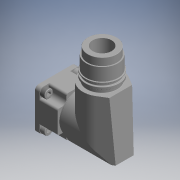
# Autodesk Inventor part: SCHUNK-Stecker ERD
Saved by Autodesk Inventor 2017.3 (Build 213256000, 256)
## iProperties
Part Number: SCHUNK-Stecker ERD
Material: Generic
Catalog Web Link: www.cadenas.de
Description: Connector-Miniature rotary unit
Vendor: SCHUNK
Document SubType Name: Modeling
Designer: partserver
Manufacturer: SCHUNK
Mass: 19.4018 g
Surface Area: 56.9329 cm^2
Volume: 19.4018 cm^3
Density: 1 g/cm^3
Appearance: PSOLRGB-192-192-192
Category: PARTsolutions
Company: SCHUNK
Title: SCHUNK-Stecker ERD
Author: Cadenas PARTsolutions
Comments: Miniature rotary unit
PSOL_IDENT_0: {$CADENAS_DATA\23d-libs\schunk\greifsysteme\drehmodule\drehmodule_elektrisch\schwenkeinheiten\miniat
PSOL_IDENT_1: ur_schwenkeinheiten\erd_stk.prj},179 {VTYP=3D},{NB=SCHUNK-Stecker ERD},{LINA=SCHUNK-Stecker ERD},{NN=
PSOL_IDENT_2: Connector},{DATE=23.04.2020 15:23:31},{GEOMDATE=04.12.2019 08:06:04},{VERSION=},{LINEID=10},{WBVAR=}
PSOL_IDENT_3: ,{WBNUMERIC=}  {NB=SCHUNK-Stecker ERD},{LINA=SCHUNK-Stecker ERD},{KT=DUMMY},{TYP=ERD}
NB: SCHUNK-Stecker ERD
NN: Connector
NT: Miniature rotary unit
NBSYN: SCHUNK-Stecker $TYP.
LINA: SCHUNK-Stecker ERD
CATALOG: SCHUNK
TYP: ERD
SUPPLIER: SCHUNK
ARTICLENO: SCHUNK-Stecker ERD
BOMINFO: SCHUNK-Stecker ERD
CREATOR: CADENAS GmbH
Autodesk Inventor part; units mm, degrees
sketch "Sketch_7" plane through (0, 0, 0) normal (1, 0, 0) x (0, 1, 0)
  line L0 (21.3, -2.9) -> (3.7, -2.9)
  arc A0 (3.7, -2.9) -> (1.7, -4.9) centre (3.7, -4.9) ccw
  line L1 (1.7, -4.9) -> (1.7, -22.5)
  arc A1 (1.7, -22.5) -> (3.7, -24.5) centre (3.7, -22.5) ccw
  line L2 (3.7, -24.5) -> (21.3, -24.5)
  arc A2 (21.3, -24.5) -> (23.3, -22.5) centre (21.3, -22.5) ccw
  line L3 (23.3, -22.5) -> (23.3, -4.9)
  arc A3 (23.3, -4.9) -> (21.3, -2.9) centre (21.3, -4.9) ccw
  constraints: 8 end point, 8 point on circle, 4 centre point
extrude "Extrusion1" add sketch "Sketch_7" against normal blind 12
sketch "Sketch_8" plane through (-12, 0, 0) normal (1, 0, 0) x (0, 0, -1)
  line L0 (0.9, -0.3) -> (26.5, -0.3)
  line L1 (26.5, -0.3) -> (26.5, 25.3)
  line L2 (26.5, 25.3) -> (0.9, 25.3)
  line L3 (0.9, 25.3) -> (0.9, -0.3)
  arc A0 (2.9, 7.4) -> (3.9, 6.4) centre (3.9, 7.4) ccw
  line L4 (3.9, 6.4) -> (5.3, 6.4)
  arc A1 (7.6, 4.1) -> (5.3, 6.4) centre (5.3, 4.1) ccw
  line L5 (7.6, 4.1) -> (7.6, 2.7)
  arc A2 (7.6, 2.7) -> (8.6, 1.7) centre (8.6, 2.7) ccw
  line L6 (8.6, 1.7) -> (18.8, 1.7)
  arc A3 (18.8, 1.7) -> (19.8, 2.7) centre (18.8, 2.7) ccw
  line L7 (19.8, 2.7) -> (19.8, 4.1)
  arc A4 (22.1, 6.4) -> (19.8, 4.1) centre (22.1, 4.1) ccw
  line L8 (22.1, 6.4) -> (23.5, 6.4)
  arc A5 (23.5, 6.4) -> (24.5, 7.4) centre (23.5, 7.4) ccw
  line L9 (24.5, 7.4) -> (24.5, 17.6)
  arc A6 (24.5, 17.6) -> (23.5, 18.6) centre (23.5, 17.6) ccw
  line L10 (23.5, 18.6) -> (22.1, 18.6)
  arc A7 (19.8, 20.9) -> (22.1, 18.6) centre (22.1, 20.9) ccw
  line L11 (19.8, 20.9) -> (19.8, 22.3)
  arc A8 (19.8, 22.3) -> (18.8, 23.3) centre (18.8, 22.3) ccw
  line L12 (18.8, 23.3) -> (8.6, 23.3)
  arc A9 (8.6, 23.3) -> (7.6, 22.3) centre (8.6, 22.3) ccw
  line L13 (7.6, 22.3) -> (7.6, 20.9)
  arc A10 (5.3, 18.6) -> (7.6, 20.9) centre (5.3, 20.9) ccw
  line L14 (5.3, 18.6) -> (3.9, 18.6)
  arc A11 (3.9, 18.6) -> (2.9, 17.6) centre (3.9, 17.6) ccw
  line L15 (2.9, 17.6) -> (2.9, 7.4)
  constraints: 32 end point, 24 point on circle, 12 centre point
extrude "Extrusion2" cut sketch "Sketch_8" along normal blind 9.5
sketch "Sketch_9" plane through (0, 0, -13.7) normal (0, 0, 1) x (1, 0, 0)
  line L0 (50, 12.5) -> (-50, 12.5)
  line L1 (-36.93, 12.5) -> (-36.93, 22.75)
  line L2 (-36.93, 22.75) -> (-12.75, 22.75)
  arc A0 (-12.75, 22.75) -> (-12.35, 22.35) centre (-12.35, 22.75) ccw
  line L3 (-12.35, 22.35) -> (-12, 22.35)
  line L4 (-12, 22.35) -> (-12, 12.5)
  line L5 (-12, 12.5) -> (-36.93, 12.5)
  constraints: 12 end point, 2 point on circle, 1 centre point
revolve "Revolution1" add sketch "Sketch_9" angle 360 about axis through (50, 12.5, -13.7) along (1, 0, 0)
sketch "Sketch_10" plane through (-36.93, 0, 0) normal (1, 0, 0) x (0, 0, -1)
  line L0 (3.3, 18.15) -> (3.3, 6.85)
  line L1 (3.3, 6.85) -> (8.5222, 3.7133)
  line L2 (8.5222, 3.7133) -> (8.5222, 21.2867)
  line L3 (8.5222, 21.2867) -> (3.3, 18.15)
  constraints: 8 end point
extrude "Extrusion3" add sketch "Sketch_10" along normal blind 24.18
sketch "Sketch_11" plane through (-24.8327, 0, 0) normal (1, 0, 0) x (0, 0, -1)
  line L0 (50.05, 12.5) -> (13.7, 12.5)
  line L1 (13.7, 12.5) -> (13.7, 22.75)
  line L2 (13.7, 22.75) -> (33.95, 22.75)
  line L3 (33.95, 22.75) -> (33.95, 20.65)
  arc A0 (33.95, 20.65) -> (34.1, 20.5) centre (34.1, 20.65) ccw
  line L4 (34.1, 20.5) -> (36.05, 20.5)
  line L5 (36.05, 20.5) -> (36.05, 21.35)
  arc A1 (36.2, 21.5) -> (36.05, 21.35) centre (36.2, 21.35) ccw
  line L6 (36.2, 21.5) -> (37.2, 21.5)
  arc A2 (37.35, 21.35) -> (37.2, 21.5) centre (37.2, 21.35) ccw
  line L7 (37.35, 21.35) -> (37.35, 20.75)
  arc A3 (37.35, 20.75) -> (37.5, 20.6) centre (37.5, 20.75) ccw
  line L8 (37.5, 20.6) -> (38.7, 20.6)
  arc A4 (38.7, 20.6) -> (38.85, 20.75) centre (38.7, 20.75) ccw
  line L9 (38.85, 20.75) -> (38.85, 21.35)
  arc A5 (39, 21.5) -> (38.85, 21.35) centre (39, 21.35) ccw
  line L10 (39, 21.5) -> (39.3, 21.5)
  arc A6 (39.45, 21.35) -> (39.3, 21.5) centre (39.3, 21.35) ccw
  line L11 (39.45, 21.35) -> (39.45, 20.9)
  line L12 (39.45, 20.9) -> (46.15, 20.9)
  line L13 (46.15, 20.9) -> (46.15, 20.25)
  line L14 (46.15, 20.25) -> (49.9, 20.25)
  arc A7 (50.05, 20.1) -> (49.9, 20.25) centre (49.9, 20.1) ccw
  line L15 (50.05, 20.1) -> (50.05, 17.5)
  line L16 (50.05, 17.5) -> (42.05, 17.5)
  line L17 (42.05, 17.5) -> (42.05, 12.5)
  line L18 (42.05, 12.5) -> (13.7, 12.5)
  constraints: 38 end point, 16 point on circle, 8 centre point
revolve "Revolution2" add sketch "Sketch_11" angle 360 about axis through (-24.8327, 12.5, -50.05) along (0, 0, -1)
sketch "Sketch_13" plane through (0, 0, -13.7) normal (0, 0, 1) x (1, 0, 0)
  line L0 (-36.8327, 17.249) -> (-36.8327, 7.751)
  line L1 (-36.8327, 7.751) -> (-30.1105, 3.7133)
  line L2 (-30.1105, 3.7133) -> (-30.1105, 21.2867)
  line L3 (-30.1105, 21.2867) -> (-36.8327, 17.249)
  constraints: 8 end point
extrude "Extrusion4" add sketch "Sketch_13" against normal blind 20.25
sketch "Sketch_12" plane through (0, 0, -3.2) normal (0, 0, 1) x (1, 0, 0)
  line L0 (-39.8327, -0.15) -> (-24.8327, -0.15)
  line L1 (-24.8327, -0.15) -> (-24.8327, 2.25)
  arc A0 (-30.1105, 3.7133) -> (-24.8327, 2.25) centre (-24.8327, 12.5) ccw
  line L2 (-30.1105, 3.7133) -> (-36.8327, 7.751)
  line L3 (-36.8327, 7.751) -> (-36.8327, 17.249)
  line L4 (-36.8327, 17.249) -> (-30.1105, 21.2867)
  arc A1 (-24.8327, 22.75) -> (-30.1105, 21.2867) centre (-24.8327, 12.5) ccw
  line L5 (-24.8327, 22.75) -> (-24.8327, 25.15)
  line L6 (-24.8327, 25.15) -> (-39.8327, 25.15)
  line L7 (-39.8327, 25.15) -> (-39.8327, -0.15)
  constraints: 16 end point, 4 point on circle, 2 centre point
extrude "Extrusion5" cut sketch "Sketch_12" against normal blind 30.6878
sketch "Sketch_14" plane through (0, 0, 0) normal (0, 1, 0) x (-1, 0, 0)
  line L0 (36.833, -43.1878) -> (36.833, -2.25)
  line L1 (36.833, -2.25) -> (34.0601, -43.1878)
  line L2 (34.0601, -43.1878) -> (36.833, -43.1878)
  constraints: 6 end point
extrude "Extrusion6" cut sketch "Sketch_14" along normal blind 30.25
sketch "Sketch_31" plane through (0, 0, -5.3) normal (0, 0, 1) x (1, 0, 0)
  line L0 (50, 20.9) -> (-50, 20.9)
  line L1 (-5, 20.9) -> (-5, 22.85)
  arc A0 (-4.7, 23.15) -> (-5, 22.85) centre (-4.7, 22.85) ccw
  line L2 (-4.7, 23.15) -> (-2.5, 23.15)
  line L3 (-2.5, 23.15) -> (-2.5, 20.9)
  line L4 (-2.5, 20.9) -> (-5, 20.9)
  constraints: 10 end point, 2 point on circle, 1 centre point
revolve "Revolution3" add sketch "Sketch_31" angle 360 about axis through (50, 20.9, -5.3) along (1, 0, 0)
sketch "Sketch_32" plane through (0, 0, -5.3) normal (0, 0, 1) x (1, 0, 0)
  line L0 (50, 4.1) -> (-50, 4.1)
  line L1 (-5, 4.1) -> (-5, 6.05)
  arc A0 (-4.7, 6.35) -> (-5, 6.05) centre (-4.7, 6.05) ccw
  line L2 (-4.7, 6.35) -> (-2.5, 6.35)
  line L3 (-2.5, 6.35) -> (-2.5, 4.1)
  line L4 (-2.5, 4.1) -> (-5, 4.1)
  constraints: 10 end point, 2 point on circle, 1 centre point
revolve "Revolution4" add sketch "Sketch_32" angle 360 about axis through (50, 4.1, -5.3) along (1, 0, 0)
sketch "Sketch_33" plane through (0, 0, -22.1) normal (0, 0, 1) x (1, 0, 0)
  line L0 (50, 20.9) -> (-50, 20.9)
  line L1 (-5, 20.9) -> (-5, 22.85)
  arc A0 (-4.7, 23.15) -> (-5, 22.85) centre (-4.7, 22.85) ccw
  line L2 (-4.7, 23.15) -> (-2.5, 23.15)
  line L3 (-2.5, 23.15) -> (-2.5, 20.9)
  line L4 (-2.5, 20.9) -> (-5, 20.9)
  constraints: 10 end point, 2 point on circle, 1 centre point
revolve "Revolution5" add sketch "Sketch_33" angle 360 about axis through (50, 20.9, -22.1) along (1, 0, 0)
sketch "Sketch_34" plane through (0, 0, -22.1) normal (0, 0, 1) x (1, 0, 0)
  line L0 (50, 4.1) -> (-50, 4.1)
  line L1 (-5, 4.1) -> (-5, 6.05)
  arc A0 (-4.7, 6.35) -> (-5, 6.05) centre (-4.7, 6.05) ccw
  line L2 (-4.7, 6.35) -> (-2.5, 6.35)
  line L3 (-2.5, 6.35) -> (-2.5, 4.1)
  line L4 (-2.5, 4.1) -> (-5, 4.1)
  constraints: 10 end point, 2 point on circle, 1 centre point
revolve "Revolution6" add sketch "Sketch_34" angle 360 about axis through (50, 4.1, -22.1) along (1, 0, 0)
sketch "Sketch_35" plane through (-5, 20.9, -22.1) normal (-1, 0, 0) x (0, 1, 0)
  line L0 (-1, -0.5774) -> (0, -1.1547)
  line L1 (0, -1.1547) -> (1, -0.5774)
  line L2 (1, -0.5774) -> (1, 0.5774)
  line L3 (1, 0.5774) -> (0, 1.1547)
  line L4 (0, 1.1547) -> (-1, 0.5774)
  line L5 (-1, 0.5774) -> (-1, -0.5774)
  constraints: 12 end point
extrude "Extrusion7" cut sketch "Sketch_35" against normal blind 2
sketch "Sketch_36" plane through (-5, 20.9, -5.3) normal (-1, 0, 0) x (0, 1, 0)
  line L0 (-1, -0.5774) -> (0, -1.1547)
  line L1 (0, -1.1547) -> (1, -0.5774)
  line L2 (1, -0.5774) -> (1, 0.5774)
  line L3 (1, 0.5774) -> (0, 1.1547)
  line L4 (0, 1.1547) -> (-1, 0.5774)
  line L5 (-1, 0.5774) -> (-1, -0.5774)
  constraints: 12 end point
extrude "Extrusion8" cut sketch "Sketch_36" against normal blind 2
sketch "Sketch_37" plane through (-5, 4.1, -22.1) normal (-1, 0, 0) x (0, 1, 0)
  line L0 (-1, -0.5774) -> (0, -1.1547)
  line L1 (0, -1.1547) -> (1, -0.5774)
  line L2 (1, -0.5774) -> (1, 0.5774)
  line L3 (1, 0.5774) -> (0, 1.1547)
  line L4 (0, 1.1547) -> (-1, 0.5774)
  line L5 (-1, 0.5774) -> (-1, -0.5774)
  constraints: 12 end point
extrude "Extrusion9" cut sketch "Sketch_37" against normal blind 2
sketch "Sketch_38" plane through (-5, 4.1, -5.3) normal (-1, 0, 0) x (0, 1, 0)
  line L0 (-1, -0.5774) -> (0, -1.1547)
  line L1 (0, -1.1547) -> (1, -0.5774)
  line L2 (1, -0.5774) -> (1, 0.5774)
  line L3 (1, 0.5774) -> (0, 1.1547)
  line L4 (0, 1.1547) -> (-1, 0.5774)
  line L5 (-1, 0.5774) -> (-1, -0.5774)
  constraints: 12 end point
extrude "Extrusion10" cut sketch "Sketch_38" against normal blind 2
ref_plane "geh_XY" through (0, 12.5, -13.7) normal (1, 0, 0) x (0, 0, -1)
ref_plane "geh_YZ" through (0, 12.5, -13.7) normal (0, 0, -1) x (0, 1, 0)
ref_plane "geh_ZX" through (0, 12.5, -13.7) normal (0, 1, 0) x (1, 0, 0)
body "Solid1"
